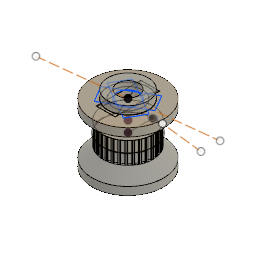
kiristingear v4 (Autodesk Fusion 360 design; units mm, degrees)
Autodesk Fusion 360 part; units mm, degrees
note: some values were not read from the file. Set by a fixed rule: which face or edge a step refers to.
sketch "Tooth Profile" plane through (0, 0, 0) normal (0, 0, 1) x (1, 0, 0)
  circle A0 centre (0, 0) radius 9.5493 construction
  circle A1 centre (0, 0) radius 9.2953
  line L0 (0, 0) -> (0, 9.5493) construction
  circle A2 centre (0, 9.1003) radius 0.555
  circle A3 centre (-0.4042, 9.2865) radius 1
  circle A4 centre (0.4042, 9.2865) radius 1
  point P0 (0, 9.2953)
  dimension "d5" = 19.0986
  dimension "d8" = 18.5906
  dimension "d10" = 0.195
  dimension "d11" = 0.555
  dimension "d30" = 1
  constraint coincident A0.centre A1.centre
  constraint coincident A0 L0.end
  constraint vertical L0
  constraint coincident L0 A2.centre
  constraint coincident A1 P0
  constraint coincident L0 P0
  constraint coincident A1 A3.centre
  constraint symmetric L0 A3 A4
  constraint tangent A2 A4
  measures "d5" diameter of A0
  measures "d8" diameter of A1
  measures "d10" distance of A2.centre P0
  measures "d11" radius of A2
  measures "d30" radius of A3
extrude "Extrude1" add sketch "Tooth Profile" along normal mid plane 8 contours A1 A3 A4 | A1 A3 A4 | A1 A3 A4 | A2 A3 A4 picked at (0.3011, -3.4158) picked at (0.8669, 8.971) picked at (-0.8669, 8.971)
fillet "Fillet1" radius 0.15 2 edges at (0.5958, 9.2762, 0) (-0.5958, 9.2762, 0)
pattern_circular "C-Pattern2" count 30 over 360 about axis through (0, 0, -4) along (0, 0, 1) of 5 faces at (-0.5584, 9.0153, 1.3333) (-0.6196, 9.214, -1.3333) (0.6196, 9.214, 1.3333) (0.5286, 8.9259, 1.3333) (-0.3821, 8.6978, 1.3333)
ref_plane "WorkPlane4" through (0, -0.0096, 4) normal (0, 0, 1) x (1, 0, 0)
sketch "Sketch12" plane through (0, 0, 4) normal (0, 0, 1) x (1, 0, 0)
  circle A0 centre (0, 0) radius 9.2953
  dimension "d99" = 18.5906
  constraint coincident A0.centre origin
  measures "d99" diameter of A0
extrude "Extrude19" add sketch "Sketch12" along normal blind 4 draft 45
extrude "Extrude20" add 1 faces at (-3.2382, 0, 8) along direction (0, 0, 1) blind 3
mirror "Mirror3" about plane through (0, 0, 0) normal (0, 0, 1) of "Extrude19", "Extrude20"
sketch "Sketch13" plane through (0, 0, 11) normal (0, 0, 1) x (-1, 0, 0)
  circle A0 centre (0, 0) radius 13.2953
  circle A1 centre (0, 0) radius 4
  circle A2 centre (0, 0) radius 7.5
  line L0 (30.831, 3.5) -> (-30.831, -3.5) construction
  line L1 (-30.7172, 3.4991) -> (-14.528, 1.6549) construction
  line L2 (-3.5, -8.2953) -> (3.5, -8.2953)
  line L3 (3.5, -8.2953) -> (3.5, 8.2953)
  line L4 (3.5, 8.2953) -> (-3.5, 8.2953)
  line L5 (-3.5, 8.2953) -> (-3.5, -8.2953)
  line L6 (-3.5, -8.2953) -> (3.5, 8.2953) construction
  line L7 (3.5, -8.2953) -> (-3.5, 8.2953) construction
  circle A3 centre (0, 0) radius 5.5493
  line L8 (-5.4339, -7.1787) -> (8.9339, 1.1166)
  line L9 (5.4339, 7.1787) -> (-8.9339, -1.1166)
  line L10 (8.9339, 1.1166) -> (5.4339, 7.1787)
  line L11 (-8.9339, -1.1166) -> (-5.4339, -7.1787)
  line L12 (8.9339, -1.1166) -> (-5.4339, 7.1787)
  line L13 (-8.9339, 1.1166) -> (5.4339, -7.1787)
  line L14 (-5.4339, 7.1787) -> (-8.9339, 1.1166)
  line L15 (5.4339, -7.1787) -> (8.9339, -1.1166)
  dimension "d107" = 8
  dimension "d108" = 15
  dimension "d109" = 7
  dimension "d110" = 17.0986
  dimension "d111" = 16.5906
  dimension "d112" = 7
  dimension "d113" = 11.0986
  dimension "d117" = 360
  constraint coincident A0.centre A1.centre
  constraint coincident L0 A0.centre
  constraint coincident L1 A0.centre
  constraint perpendicular L2 L3
  constraint parallel L2 L4
  constraint parallel L3 L5
  constraint horizontal L2
  constraint coincident L6 A0.centre
  constraint coincident L7 A0.centre
  measures "d107" diameter of A1
  measures "d108" diameter of A2
  measures "d109" distance of L1.start L0.end
  measures "d110" distance of L0.end L1.end
  measures "d111" distance of L2.end L3.end
  measures "d112" distance of L3.end L4.end
  measures "d113" diameter of A3
extrude "Extrude32" cut sketch "Sketch13" against normal up to surface (22 mm away) contours A1 L3 | A1 L3 L5 L8 L9 L12 L13 | A1 L12 | A1 L8 | A1 L9 | A1 L13 | A1 L5
extrude "Extrude33" add sketch "Sketch13" along normal blind 3 contours A1 L3 A3 L8 L12 | A1 L3 L12 | A1 L3 L8 | A1 L3 A3 L9 L12 | L3 A3 L12 | A1 L3 A3 L8 L13 | L3 A3 L8 | A1 L9 L12 | L3 A3 L9 | A2 L3 A3 L8 L9 L12 | A3 L8 L12 | A1 L8 L13 | A2 L3 A3 L8 L12 L13 | L3 A3 L13 | A1 L5 A3 L9 L12 | A3 L9 L12 | A2 L3 L5 A3 L9 L12 | A2 L3 L9 | A2 L8 L12 | A1 L5 A3 L8 L13 | A3 L8 L13 | A2 L3 L13 | A2 L3 L5 A3 L8 L13 | A1 L5 L9 | L5 A3 L12 | A1 L5 L13 | L5 A3 L8 | A1 L5 A3 L9 L13 | L5 A3 L9 | A2 L5 A3 L9 L12 L13 | A2 L5 L12 | L5 A3 L13 | A2 L5 A3 L8 L9 L13 | A2 L5 L8 | A3 L9 L13 | A2 L9 L13
equation "numTeeth = 30"
equation "pitch = 2 mm"
equation "pi = 3.14159"
equation "pulleyPitchDiam = ( numTeeth * pitch ) / pi"
equation "d5 = pulleyPitchDiam"
equation "pitchLineDifferential = 0.254 mm"
equation "pulleyOuterDiameter = pulleyPitchDiam - ( 2 * pitchLineDifferential )"
equation "d8 = pulleyOuterDiameter"
equation "d10 = 0.75 mm - 0.555 mm"
equation "d14 = pulleyWidth"
equation "d33 = numTeeth"
equation "flangeHeight = 4 mm"
equation "adapterDiameter = 20 mm"
equation "adapterHeight = 10 mm"
equation "pulleyWidth = 8 mm"
equation "topHeight = 1.6 mm"
equation "motorShaftBore = 5.5 mm"
equation "setScrewHeight = 0.5"
equation "motorShaftDepth = 8 mm"
equation "setScrewDiam = 3 mm"
equation "d99 = pulleyOuterDiameter"
equation "d100 = flangeHeight"
equation "hole_diam = 8 mm"
equation "d107 = hole_diam"
equation "d108 = hole_diam + 7 mm"
equation "d110 = pulleyPitchDiam - 2 mm"
equation "d111 = pulleyOuterDiameter - 2 mm"
equation "d113 = pulleyPitchDiam - 8 mm"
